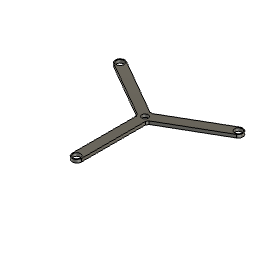
Spectroscope Mount v1 (Autodesk Fusion 360 design; units mm, degrees)
Autodesk Fusion 360 part; units mm, degrees
sketch "Sketch1" plane through (0, 0, 0) normal (0, 0, 1) x (1, 0, 0) in component "Spectroscope Feet"
  circle A0 centre (96.1288, 55.5) radius 6
  circle A1 centre (-96.1288, 55.5) radius 6
  circle A2 centre (0, -111) radius 6
  circle A3 centre (0, -111) radius 7.5
  circle A4 centre (-96.1288, 55.5) radius 7.5
  circle A5 centre (96.1288, 55.5) radius 7.5
  circle A6 centre (0, 0) radius 10
  line L0 (92.3788, 61.9952) -> (1.9782, 9.8024)
  line L1 (99.8788, 49.0048) -> (9.4782, -3.188)
  line L2 (-99.8788, 49.0048) -> (-9.4782, -3.188)
  line L3 (-92.3788, 61.9952) -> (-1.9782, 9.8024)
  line L4 (-7.5, -111) -> (-7.5, -6.6144)
  line L5 (7.5, -111) -> (7.5, -6.6144)
  circle A7 centre (0, 0) radius 5
  dimension "d4" = 12
  dimension "d5" = 12
  dimension "d6" = 12
  dimension "d7" = 15
  dimension "d8" = 15
  dimension "d9" = 15
  dimension "d10" = 20
  dimension "d11" = 10
  constraint concentric A2 A3
  constraint concentric A1 A4
  constraint concentric A0 A5
  constraint coincident A6.centre A7.centre
  constraint coincident A5 L1.start
  constraint coincident A5 L0.start
  constraint coincident A6 L0.end
  constraint tangent A5 L0
  constraint coincident A6 L1.end
  constraint tangent A5 L1
  constraint coincident A4 L3.start
  constraint coincident A4 L2.start
  constraint coincident A6 L2.end
  constraint tangent A4 L2
  constraint coincident A6 L3.end
  constraint tangent A4 L3
  constraint coincident A3 L5.start
  constraint coincident A3 L4.start
  constraint coincident A6 L4.end
  constraint tangent A3 L4
  constraint coincident A6 L5.end
  constraint tangent A3 L5
  measures "d4" diameter of A0
  measures "d5" diameter of A1
  measures "d6" diameter of A2
  measures "d7" diameter of A3
  measures "d8" diameter of A4
  measures "d9" diameter of A5
  measures "d10" diameter of A6
  measures "d11" diameter of A7
extrude "Extrude1" add sketch "Sketch1" along normal blind 5 in component "Spectroscope Feet"
component "Spectroscope Feet" placed x (1, 0, 0) y (0, 1, 0) z (0, 0, 1) at (0, 0, 0)
